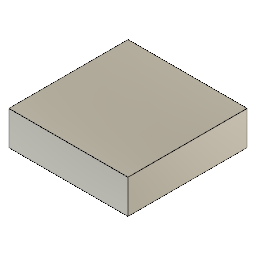
net_mk5 v34 (Autodesk Fusion 360 archive; units mm, degrees)
design "Wyse 3040"
Autodesk Fusion 360 part; units mm, degrees
sketch "Sketch1" plane through (0, 0, 0) normal (0, 0, 1) x (1, 0, 0)
  line L0 (0, 0) -> (101.5, 0)
  line L1 (101.5, 0) -> (101.5, 101.5)
  line L2 (101.5, 101.5) -> (0, 101.5)
  line L3 (0, 101.5) -> (0, 0)
  dimension "d1" = 101.5
  dimension "d2" = 101.5
  constraint horizontal L0
  constraint vertical L1
  constraint horizontal L2
  constraint vertical L3
  constraint coincident L0.start L3.end
  measures "d1" distance of L1.end L2.end
  measures "d2" distance of L0.end L1.end
extrude "Extrude1" add sketch "Sketch1" along normal blind 29
equation "d2 = d1"
